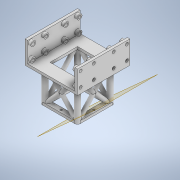
# Autodesk Inventor part: gantry3
Saved by Autodesk Inventor 2022 (Build 260153000, 153)
## iProperties
Created: 2022-03-29
Part Number: gantry3
Material: Generic
Document SubType Name: Modeling
Designer: Phabryan
Density: 1 g/cm^3
Appearance: Default
Author: Phabryan
Autodesk Inventor part; units mm, degrees
ref_plane "YZ Plane" through (0, 0, 0) normal (1, 0, 0) x (0, 1, 0)
ref_plane "XZ Plane" through (0, 0, 0) normal (0, 1, 0) x (-1, 0, 0)
ref_plane "XY Plane" through (0, 0, 0) normal (0, 0, 1) x (1, 0, 0)
sketch "Sketch1" plane through (0, 0, 0) normal (0, 1, 0) x (-1, 0, 0)
  line L0 (51.5, 51.5) -> (-51.5, 51.5)
  line L1 (-51.5, 51.5) -> (-51.5, -51.5)
  line L2 (-51.5, -51.5) -> (51.5, -51.5)
  line L3 (51.5, -51.5) -> (51.5, 51.5)
  point P0 (0, 0)
  dimension "d0" = 103
  dimension "d1" = 103
  constraints: 8 end point, 2 parallel, 1 horizontal, 1 perpendicular
  measures "d0" distance of L2.end L1.end
  measures "d1" distance of L1.end L0.end
extrude "Extrusion1" add sketch "Sketch1" along normal blind 5
sketch "Sketch2" plane through (0, 5, 0) normal (0, 1, 0) x (1, 0, 0)
  line L0 (-51.5, 51.5) -> (-51.5, -51.5) projected
  line L1 (-51.5, -51.5) -> (-46.5, -51.5)
  line L2 (-46.5, -51.5) -> (-46.5, 51.5)
  line L3 (-46.5, 51.5) -> (-51.5, 51.5)
  line L4 (-51.5, 51.5) -> (-51.5, -51.5)
  line L5 (51.5, 51.5) -> (-51.5, 51.5) projected
  line L6 (-51.5, -51.5) -> (51.5, -51.5) projected
  line L7 (51.5, 51.5) -> (46.5, 51.5)
  line L8 (46.5, 51.5) -> (46.5, -51.5)
  line L9 (46.5, -51.5) -> (51.5, -51.5)
  line L10 (51.5, -51.5) -> (51.5, 51.5)
  point P0 (0, 0)
  dimension "d4" = 5
  dimension "d5" = 5
  constraints: 16 end point, 4 parallel, 2 horizontal, 2 perpendicular, 1 point on line
  measures "d4" distance of L3.end L2.end
  measures "d5" distance of L9.end L8.end
extrude "Extrusion2" add sketch "Sketch2" along normal blind 40 contours L3 L2 L1 L0 | L5 L10 L6 L8
sketch "Sketch3" plane through (-46.5, 5, 51.5) normal (1, 0, 0) x (0, 0, -1)
  circle A0 centre (6, 34) radius 5
  circle A1 centre (6, 6) radius 5
  circle A2 centre (97, 34) radius 5
  circle A3 centre (97, 6) radius 5
  circle A4 centre (32, 34) radius 5
  circle A5 centre (32, 6) radius 5
  circle A6 centre (71, 34) radius 5
  circle A7 centre (71, 6) radius 5
  circle A8 centre (6, 34) radius 3
  circle A9 centre (6, 6) radius 3
  circle A10 centre (32, 34) radius 3
  circle A11 centre (32, 6) radius 3
  circle A12 centre (71, 34) radius 3
  circle A13 centre (71, 6) radius 3
  circle A14 centre (97, 34) radius 3
  circle A15 centre (97, 6) radius 3
  point P0 (51.5, -5)
  dimension "d8" = 10
  dimension "d9" = 10
  dimension "d10" = 10
  dimension "d11" = 10
  dimension "d12" = 10
  dimension "d13" = 10
  dimension "d14" = 10
  dimension "d15" = 10
  dimension "d16" = 6
  dimension "d17" = 6
  dimension "d18" = 6
  dimension "d19" = 6
  dimension "d20" = 6
  dimension "d21" = 6
  dimension "d22" = 6
  dimension "d23" = 6
  constraints: 16 centre point, 8 coincident
  measures "d8" diameter of A0
  measures "d9" diameter of A1
  measures "d10" diameter of A2
  measures "d11" diameter of A3
  measures "d12" diameter of A4
  measures "d13" diameter of A5
  measures "d14" diameter of A6
  measures "d15" diameter of A7
  measures "d16" diameter of A8
  measures "d17" diameter of A9
  measures "d18" diameter of A10
  measures "d19" diameter of A11
  measures "d20" diameter of A12
  measures "d21" diameter of A13
  measures "d22" diameter of A14
  measures "d23" diameter of A15
extrude "Extrusion3" add sketch "Sketch3" along normal blind 5 contours A0 | A1 | A2 | A3 | A4 | A5 | A6 | A7 | A8 | A9 | A10 | A11 | A12 | A13 | A14 | A15
sketch "Sketch4" plane through (-41.5, 39, 45.5) normal (1, 0, 0) x (0, 0, -1)
  circle A0 centre (0, 0) radius 5 projected
  circle A1 centre (0, 0) radius 3
  circle A2 centre (0, -28) radius 5 projected
  circle A3 centre (0, -28) radius 3
  circle A4 centre (26, 0) radius 5 projected
  circle A5 centre (26, 0) radius 3
  circle A6 centre (26, -28) radius 5 projected
  circle A7 centre (26, -28) radius 3
  circle A8 centre (65, 0) radius 5 projected
  circle A9 centre (65, 0) radius 3
  circle A10 centre (65, -28) radius 5 projected
  circle A11 centre (65, -28) radius 3
  circle A12 centre (91, 0) radius 5 projected
  circle A13 centre (91, 0) radius 3
  circle A14 centre (91, -28) radius 5 projected
  circle A15 centre (91, -28) radius 3
  point P0 (45.5, -39)
  dimension "d26" = 6
  dimension "d27" = 6
  dimension "d28" = 6
  dimension "d29" = 6
  dimension "d30" = 6
  dimension "d31" = 6
  dimension "d32" = 6
  dimension "d33" = 6
  constraints: 8 centre point, 8 coincident
  measures "d26" diameter of A1
  measures "d27" diameter of A3
  measures "d28" diameter of A5
  measures "d29" diameter of A7
  measures "d30" diameter of A9
  measures "d31" diameter of A11
  measures "d32" diameter of A13
  measures "d33" diameter of A15
extrude "Extrusion4" cut sketch "Sketch4" against normal blind 20 contours A1 | A3 | A5 | A7 | A9 | A11 | A13 | A15
mirror "Mirror1" about plane through (0, 0, 0) normal (1, 0, 0) of "Extrusion4", "Extrusion3"
sketch "Sketch5" plane through (0, 0, 0) normal (0, -1, 0) x (1, 0, 0)
  circle A0 centre (32, 32) radius 5
  circle A1 centre (32, -32) radius 5
  circle A2 centre (-32, -32) radius 5
  circle A3 centre (-32, 32) radius 5
  point P0 (0, 0)
  dimension "d36" = 10
  dimension "d37" = 10
  dimension "d38" = 10
  dimension "d39" = 10
  constraints: 4 centre point
  measures "d36" diameter of A0
  measures "d37" diameter of A1
  measures "d38" diameter of A2
  measures "d39" diameter of A3
extrude "Extrusion5" add sketch "Sketch5" along normal blind 65
sketch "Sketch6" plane through (32, -65, 32) normal (0, -1, 0) x (1, 0, 0)
  circle A0 centre (-64, -64) radius 5 projected
  line L0 (-64, -69) -> (0, -69)
  circle A1 centre (0, -64) radius 5 projected
  line L1 (5, -64) -> (5, 0)
  circle A2 centre (0, 0) radius 5 projected
  line L2 (0, 5) -> (-64, 5)
  circle A3 centre (-64, 0) radius 5 projected
  line L3 (-69, 0) -> (-69, -64)
  point P0 (-32, -32)
  constraints: 8 end point, 7 point on circle, 3 tangent, 2 horizontal
extrude "Extrusion6" add sketch "Sketch6" against normal blind 5
sketch "Sketch7" plane through (0, -65, 0) normal (0, -1, 0) x (1, 0, 0)
  line L0 (27, 27) -> (-27, 27)
  line L1 (-27, 27) -> (-27, -27)
  line L2 (-27, -27) -> (27, -27)
  line L3 (27, -27) -> (27, 27)
  point P0 (0, 0)
  dimension "d44" = 54
  dimension "d45" = 54
  constraints: 8 end point, 2 parallel, 1 horizontal, 1 perpendicular
  measures "d44" distance of L2.end L1.end
  measures "d45" distance of L1.end L0.end
extrude "Extrusion7" cut sketch "Sketch7" against normal blind 100
sketch "Sketch8" plane through (0, -65, 0) normal (0, -1, 0) x (1, 0, 0)
  circle A0 centre (-32, 0) radius 2
  point P0 (0, 0)
  dimension "d48" = 4
  constraints: 1 centre point
  measures "d48" diameter of A0
extrude "Extrusion8" cut sketch "Sketch8" against normal blind 6
pattern_circular "Circular Pattern1" count 4 over 360 about axis through (0, -10, 0) along (0, 1, 0) of "Extrusion8"
ref_plane "Work Plane1" through (27, -60, 13.5) normal (-0.6691306, 0.7431448, 0) x (0, 0, 1)
sketch "Sketch9" plane through (27, -60, 13.5) normal (-0.6691306, 0.7431448, 0) x (0, 0, 1)
  ellipse E0 centre (-45.5, 3.7157) end of major axis (-50.5, 3.7157) minor radius 3.7157 (-50.5, 3.7157) -> (-45.5, 7.4314) ccw projected
  circle A0 centre (-45.5, 0) radius 3.75
  point P0 (-13.5, 20.0829)
  dimension "d55" = 7.5
  constraints: 1 centre point, 2 other
  measures "d55" diameter of A0
extrude "Extrusion9" add sketch "Sketch9" along normal blind 83 and the other way blind 2
mirror "Mirror2" about plane through (0, 0, 0) normal (1, 0, 0) of "Extrusion9"
pattern_circular "Circular Pattern2" count 4 over 360 about axis through (0, -10, 0) along (0, 1, 0) of "Extrusion9", "Mirror2"
body "Solid1"
